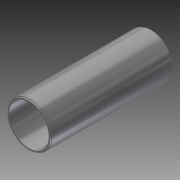
# Autodesk Inventor part: Accumulator Body Tube
Saved by Autodesk Inventor 2014 SP1 (Build 180222100, 222)
## iProperties
Category: Pneumatics
Created: 2007-11-13
Document SubType Name: Modeling
Density: 8.08 g/cm^3
Material: Stainless Steel
Description: Accumulator Body Tube
Vendor: Clippard
Mass: 463.555 g
Surface Area: 462.724 cm^2
Volume: 57.3706 cm^3
Project: FIRST
Appearance: Stainless - Brushed
Title: Accumulator Body Tube
Author: Autodesk, Inc.
Autodesk Inventor part; units mm, degrees
ref_plane "YZ Plane" through (0, 0, 0) normal (1, 0, 0) x (0, 1, 0)
ref_plane "XZ Plane" through (0, 0, 0) normal (0, 1, 0) x (-1, 0, 0)
ref_plane "XY Plane" through (0, 0, 0) normal (0, 0, 1) x (1, 0, 0)
sketch "Sketch1" plane through (0, 0, 0) normal (0, 0, 1) x (1, 0, 0)
  circle A0 centre (0, 0) radius 26.1874
  circle A1 centre (0, 0) radius 23.6474
  dimension "d0" = 52.3748
  dimension "d1" = 2.54
  constraints: 2 centre point, 2 coincident
  measures "d0" diameter of A0
  measures "d1" radial gap between concentric circles of A0 A1
extrude "Extrusion1" add sketch "Sketch1" along normal mid plane 145.288
sketch "Sketch2" plane through (0, 0, 0) normal (1, 0, 0) x (0, 1, 0)
  line L0 (-26.1874, 72.644) -> (26.1874, 72.644) projected
  line L1 (-23.6474, 72.644) -> (23.6474, 72.644) projected
  line L2 (26.1874, 72.644) -> (25.4, 72.644)
  line L3 (25.4, 72.644) -> (25.4, 71.0565)
  line L4 (25.4, 71.0565) -> (26.1874, 71.0565)
  line L5 (26.1874, 71.0565) -> (26.1874, 72.644)
  line L6 (0, -14.5288) -> (0, 87.1728) projected
  point P0 (0, 0)
  dimension "d4" = 1.5875
  dimension "d5" = 0.7874
  constraints: 8 end point, 2 parallel, 1 horizontal, 1 perpendicular
  measures "d4" distance of L4.end L0.end
  measures "d5" distance of L3.end L4.end
revolve "Revolution1" cut sketch "Sketch2" angle 360 about axis through (0, 0, -10) along (0, 0, 1)
mirror "Mirror1" about plane through (0, 0, 0) normal (0, 0, 1) of "Revolution1"
body "Solid1"
